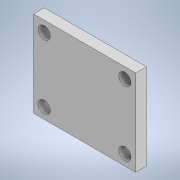
# Autodesk Inventor part: RD004
Saved by Autodesk Inventor 2021 (Build 250183000, 183)
## iProperties
Created: 2020-10-26
Part Number: RD004
Material: 一般
Document SubType Name: Modeling
Designer: ryusei
Density: 1 g/cm^3
Appearance: 既定
Author: ryusei
Title: スペーサ
Autodesk Inventor part; units mm, degrees
ref_plane "YZ Plane" through (0, 0, 0) normal (1, 0, 0) x (0, 1, 0)
ref_plane "XZ Plane" through (0, 0, 0) normal (0, 1, 0) x (-1, 0, 0)
ref_plane "XY Plane" through (0, 0, 0) normal (0, 0, 1) x (1, 0, 0)
sketch "スケッチ1" plane through (0, 0, 0) normal (0, 0, 1) x (1, 0, 0)
  line L0 (0, 0) -> (38, 0)
  line L1 (38, 0) -> (38, 32)
  line L2 (38, 32) -> (0, 32)
  line L3 (0, 32) -> (0, 0)
  dimension "d0" = 38
  dimension "d1" = 32
  constraints: 8 end point, 2 parallel, 1 horizontal, 1 perpendicular
  measures "d0" distance between parallel lines of L1 L3
  measures "d1" distance between parallel lines of L0 L2
extrude "押し出し1" add sketch "スケッチ1" along normal blind 4
sketch "スケッチ2" plane through (0, 0, 4) normal (0, 0, 1) x (1, 0, 0)
  line L0 (38, 32) -> (0, 32) projected
  line L1 (0, 32) -> (0, 0) projected
  point P0 (4, 28)
  point P1 (4, 4)
  point P2 (34, 28)
  point P3 (34, 4)
  dimension "d4" = 4
  dimension "d5" = 4
  dimension "d8" = 24
  dimension "d11" = 30
  constraints: 1 horizontal, 1 vertical, 3 other
  measures "d4" distance from line of L0 point (4, 28)
  measures "d5" distance from line of L1 point (4, 28)
  measures "d8" distance of point (4, 28) point (4, 4)
  measures "d11" distance of point (4, 28) point (34, 28)
hole "穴1" at (4, 28, 4) at (4, 4, 4) at (34, 28, 4) at (34, 4, 4) direction (0, 0, -1) diameter 4.5 end through all
